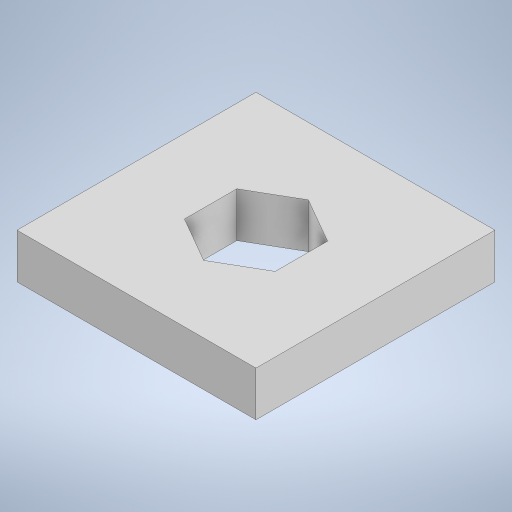
# Autodesk Inventor part: Hex Box +4mm
Saved by Autodesk Inventor 2023 (Build 270158000, 158)
## iProperties
Created: 2023-01-21
Part Number: Hex Box +4mm
Material: Generic
Document SubType Name: Modeling
Designer: bugme
Density: 1 g/cm^3
Appearance: Default
Author: bugme
Autodesk Inventor part; units mm, degrees
ref_plane "YZ Plane" through (0, 0, 0) normal (1, 0, 0) x (0, 1, 0)
ref_plane "XZ Plane" through (0, 0, 0) normal (0, 1, 0) x (-1, 0, 0)
ref_plane "XY Plane" through (0, 0, 0) normal (0, 0, 1) x (1, 0, 0)
sketch "Sketch1" plane through (0, 0, 0) normal (0, 1, 0) x (-1, 0, 0)
  line L0 (9.7983, 4.6669) -> (9.7983, -46.1331)
  line L1 (9.7983, -46.1331) -> (-41.0017, -46.1331)
  line L2 (-41.0017, -46.1331) -> (-41.0017, 4.6669)
  line L3 (-41.0017, 4.6669) -> (9.7983, 4.6669)
  line L4 (-15.6017, -31.8664) -> (-25.2435, -26.2998)
  line L5 (-25.2435, -26.2998) -> (-25.2435, -15.1664)
  line L6 (-25.2435, -15.1664) -> (-15.6017, -9.5998)
  line L7 (-15.6017, -9.5998) -> (-5.96, -15.1664)
  line L8 (-5.96, -15.1664) -> (-5.96, -26.2998)
  line L9 (-5.96, -26.2998) -> (-15.6017, -31.8664)
  point P0 (0, 0)
  point P1 (-15.6017, -20.7331)
  point P2 (-20.4226, -29.0831)
  point P3 (-10.7809, -12.3831)
  dimension "d0" = 50.8
  dimension "d1" = 50.8
  dimension "d2" = 16.7
  constraints: 20 end point, 3 perpendicular, 2 midpoint, 1 vertical, 13 other
  measures "d0" distance of L0.start L0.end
  measures "d1" distance of L0.end L1.end
  measures "d2" vertical distance of point (-20.423, -29.083) point (-10.781, -12.383)
extrude "Extrusion1" add sketch "Sketch1" along normal blind 9.525
body "Solid1"
